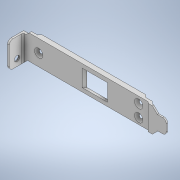
# Autodesk Inventor part: pcie-bracket
Saved by Autodesk Inventor 2021 (Build 250183000, 183)
## iProperties
Created: 2024-03-16
Part Number: pcie-bracket
Material: Generic
Document SubType Name: Modeling
Designer: Toby
Density: 1 g/cm^3
Appearance: Default
Author: Toby
Autodesk Inventor part; units mm, degrees
ref_plane "YZ Plane" through (0, 0, 0) normal (1, 0, 0) x (0, 1, 0)
ref_plane "XZ Plane" through (0, 0, 0) normal (0, 1, 0) x (-1, 0, 0)
ref_plane "XY Plane" through (0, 0, 0) normal (0, 0, 1) x (1, 0, 0)
sketch "Sketch1" plane through (0, 0, 0) normal (0, 0, 1) x (1, 0, 0)
  line L0 (-54.464, 10.0328) -> (58.286, 10.0328)
  line L1 (58.286, 10.0328) -> (58.286, -10.415)
  line L2 (58.286, -10.415) -> (-54.464, -10.415)
  line L3 (-54.464, -10.415) -> (-54.464, 10.0328)
  line L4 (58.286, 5.794) -> (65.556, 5.794)
  line L5 (65.556, 5.794) -> (65.556, -5.8813)
  line L6 (65.556, -5.8813) -> (58.286, -5.8813)
  line L7 (58.286, -5.8813) -> (58.286, 5.794)
  point P0 (0, 0)
  dimension "d0" = 112.75
  dimension "d1" = 120.02
  constraints: 16 end point, 4 parallel, 2 horizontal, 2 perpendicular, 1 point on line
  measures "d0" distance of L0.start L0.end
  measures "d1" distance between parallel lines of L3 L5
extrude "Extrusion1" add sketch "Sketch1" along normal blind 2
chamfer "Chamfer1" distance 4.2 angle 45 2 edges at (58.286, 10.0328, 1) (58.286, -10.415, 1)
fillet "Fillet1" radius 2 2 edges at (65.556, 5.794, 1) (65.556, -5.8813, 1)
sketch "Sketch3" plane through (-54.464, -10.415, 0) normal (-1, 0, 0) x (0, 0, 1)
  line L0 (0, 20.4479) -> (0, 0) projected
  line L1 (0, 17.9079) -> (13.43, 17.9079)
  line L2 (13.43, 17.9079) -> (13.43, -3.6821)
  line L3 (13.43, -3.6821) -> (0, -3.6821)
  line L4 (0, -3.6821) -> (0, 17.9079)
  line L5 (0, 20.4479) -> (2, 20.4479) projected
  line L6 (2, 20.4479) -> (2, 0) projected
  point P0 (0, 10.415)
  dimension "d14" = 2.54
  dimension "d15" = 21.59
  dimension "d16" = 11.43
  constraints: 8 end point, 2 parallel, 1 horizontal, 1 perpendicular, 1 point on line
  measures "d14" distance between parallel lines of L5 L1
  measures "d15" distance of L1.end L2.end
  measures "d16" distance between parallel lines of L2 L6
extrude "Extrusion3" add sketch "Sketch3" along normal blind 1.5 contours L1 L2 L3 L4 L0
sketch "Sketch4" plane through (0, 0, 0) normal (0, 0, -1) x (-1, 0, 0)
  line L0 (55.964, -14.0972) -> (55.964, 7.4928) projected
  line L1 (-54.086, 10.0328) -> (54.464, 10.0328) projected
  line L2 (55.964, 7.4928) -> (52.024, 7.4928)
  line L3 (52.024, 7.4928) -> (52.024, 10.0328)
  line L4 (52.024, 10.0328) -> (55.964, 10.0328)
  line L5 (55.964, 10.0328) -> (55.964, 7.4928)
  point P0 (0, 0)
  point P1 (-30.556, 10.0328)
  dimension "d19" = 3.94
  constraints: 8 end point, 2 parallel, 1 horizontal, 1 perpendicular, 1 point on line
  measures "d19" distance between parallel lines of L3 L5
extrude "Extrusion4" cut sketch "Sketch4" against normal blind 20
chamfer "Chamfer3" distance 2.54 angle 45 1 edges at (-52.024, 10.0328, 1)
chamfer "Chamfer4" distance 3.68 angle 45 1 edges at (-54.464, -10.415, 1)
fillet "Fillet2" radius 3 2 edges at (-55.214, 7.4928, 13.43) (-55.214, -14.0972, 13.43)
sketch "Sketch5" plane through (-55.964, -10.415, 0) normal (-1, 0, 0) x (0, 0, 1)
  circle A0 centre (7.08, 2.0279) radius 2.21
  line L0 (0, -3.6821) -> (10.43, -3.6821) projected
  line L1 (9.29, 2.0279) -> (4.87, 2.0279)
  line L2 (4.87, 2.0279) -> (4.87, -3.6821)
  line L3 (4.87, -3.6821) -> (9.29, -3.6821)
  line L4 (9.29, -3.6821) -> (9.29, 2.0279)
  line L5 (2, 20.4479) -> (0, 20.4479) projected
  line L6 (2, 17.9079) -> (2, 20.4479) projected
  point P0 (0, 10.415)
  point P1 (7.08, 2.0279)
  point P2 (9.29, -3.6821)
  point P3 (4.87, 2.0279)
  dimension "d29" = 4.42
  dimension "d30" = 18.42
  dimension "d31" = 5.08
  dimension "d32" = 5.08
  dimension "d33" = 4.42
  constraints: 8 end point, 2 parallel, 1 coincident, 1 horizontal, 1 midpoint, 1 perpendicular, 1 point on line, 3 other
  measures "d30" distance from line of L5 point (7.08, 2.028)
  measures "d31" distance from line of L6 point (7.08, 2.028)
  measures "d32" distance from line of L6 point (7.08, 2.028)
  measures "d33" distance between parallel lines of L2 L4
extrude "Extrusion5" cut sketch "Sketch5" against normal blind 2
fillet "Fillet3" radius 1 1 edges at (-54.464, -3.3011, 2)
fillet "Fillet4" radius 1 1 edges at (-55.964, -3.3022, 0)
sketch "Sketch13" plane through (0, 0, 0) normal (0, 0, -1) x (-1, 0, 0)
  line L0 (-1.036, 6.4328) -> (0.964, 6.4328)
  line L1 (0.964, 6.4328) -> (-0.036, 8.0328)
  line L2 (-0.036, 8.0328) -> (-1.036, 6.4328)
  line L3 (-54.086, 10.0328) -> (49.484, 10.0328) projected
  line L4 (54.964, 7.4928) -> (54.964, -14.0972) projected
  point P0 (0, 0)
  point P1 (-30.556, 10.0328)
  dimension "d84" = 2
  dimension "d85" = 1.6
  dimension "d86" = 1
  dimension "d87" = 2
  dimension "d88" = 55
  constraints: 6 end point, 1 horizontal
  measures "d84" distance of L0.end L0.start
  measures "d85" vertical distance of L0.end L1.end
  measures "d86" horizontal distance of L0.start L1.end
  measures "d87" distance from line of L3 L1.end
  measures "d88" distance from line of L4 L1.end
extrude "Extrusion12" cut sketch "Sketch13" against normal blind 0.4
sketch "Sketch14" plane through (0, 0, 2) normal (0, 0, 1) x (1, 0, 0)
  line L0 (-54.464, -11.0972) -> (-54.464, 4.4928) projected
  line L1 (-50.784, -10.415) -> (54.086, -10.415) projected
  line L2 (54.086, 10.0328) -> (-49.484, 10.0328) projected
  point P0 (0, 0)
  point P1 (-41.464, -0.415)
  point P2 (41.536, -5.415)
  point P3 (41.536, 4.585)
  dimension "d91" = 13
  dimension "d92" = 10
  dimension "d93" = 96
  dimension "d94" = 96
  dimension "d95" = 15
  dimension "d96" = 5
  dimension "d97" = 5.4479
  measures "d91" distance from line of L0 point (-41.464, -0.415)
  measures "d92" distance from line of L1 point (-41.464, -0.415)
  measures "d93" distance from line of L0 point (41.536, 4.585)
  measures "d94" distance from line of L0 point (41.536, -5.415)
  measures "d95" distance from line of L1 point (41.536, 4.585)
  measures "d96" distance from line of L1 point (41.536, -5.415)
  measures "d97" distance from line of point (41.536, 4.585) L2
hole "Hole2" at (-41.464, -0.415, 2) at (41.536, -5.415, 2) at (41.536, 4.585, 2) direction (0, 0, -1) diameter 3 depth 5 tip angle 118 countersink diameter 7 countersink angle 90
sketch "Sketch17" plane through (-49.484, 10.0328, 0) normal (0, 1, 0) x (1, 0, 0)
  line L0 (103.57, -2) -> (0, -2) projected
  line L1 (5.02, -2) -> (100.04, -2)
  line L2 (100.04, -2) -> (100.04, 2)
  line L3 (100.04, 2) -> (5.02, 2)
  line L4 (5.02, 2) -> (5.02, -2)
  line L5 (-4.98, -10.43) -> (-4.98, -3) projected
  line L6 (115.04, -2) -> (115.04, 0) projected
  point P0 (49.484, 0)
  dimension "d114" = 4
  dimension "d115" = 10
  dimension "d116" = 15
  constraints: 8 end point, 2 parallel, 1 horizontal, 1 perpendicular, 1 point on line
  measures "d114" distance between parallel lines of L0 L3
  measures "d115" distance between parallel lines of L5 L4
  measures "d116" distance from line of L6 L2.end
extrude "Extrusion14" add sketch "Sketch17" against normal blind 1.2
chamfer "Chamfer8" distance 2 angle 45 2 edges at (-44.464, 9.4328, -2) (50.556, 9.4328, -2)
sketch "Sketch18" plane through (0, 0, 2) normal (0, 0, 1) x (1, 0, 0)
  line L0 (-3.464, 6.385) -> (13.536, 6.385)
  line L1 (13.536, 6.385) -> (13.536, -6.815)
  line L2 (13.536, -6.815) -> (-3.464, -6.815)
  line L3 (-3.464, -6.815) -> (-3.464, 6.385)
  circle A0 centre (41.536, 4.585) radius 1.5 projected
  line L4 (-50.784, -10.415) -> (54.086, -10.415) projected
  point P0 (0, 0)
  dimension "d122" = 28
  dimension "d123" = 45
  dimension "d124" = 3.6
  dimension "d125" = 13.2
  constraints: 8 end point, 2 parallel, 1 horizontal, 1 perpendicular
  measures "d122" distance from line of A0.centre L1
  measures "d123" distance from line of A0.centre L3
  measures "d124" distance between parallel lines of L4 L2
  measures "d125" distance between parallel lines of L2 L0
extrude "Extrusion15" cut sketch "Sketch18" against normal blind 2 contours L0 L1 L2 L3
sketch "Sketch20" plane through (0, 0, 2) normal (0, 0, 1) x (1, 0, 0)
  line L0 (65.556, -5.8813) -> (58.286, -5.8813)
  line L1 (58.286, -5.8813) -> (58.286, 5.794)
  line L2 (58.286, 5.794) -> (65.556, 5.794)
  line L3 (65.556, 5.794) -> (65.556, -5.8813)
  line L4 (58.286, -10.415) -> (51.286, -10.415)
  line L5 (51.286, -10.415) -> (51.286, 10.0328)
  line L6 (51.286, 10.0328) -> (58.286, 10.0328)
  line L7 (58.286, 10.0328) -> (58.286, -10.415)
  line L8 (65.556, -3.8813) -> (65.556, 3.794) projected
  line L9 (58.286, -5.8813) -> (63.556, -5.8813) projected
  line L10 (63.556, 5.794) -> (58.286, 5.794) projected
  line L11 (54.086, 10.0328) -> (-49.484, 10.0328) projected
  line L12 (-50.784, -10.415) -> (54.086, -10.415) projected
  line L13 (58.286, -6.215) -> (58.286, -5.8813) projected
  point P0 (0, 0)
  dimension "d136" = 7
  constraints: 16 end point, 6 collinear, 4 parallel, 2 horizontal, 2 perpendicular, 1 point on line
  measures "d136" distance of L4.start L4.end
extrude "Extrusion17" add sketch "Sketch20" along normal blind 2
chamfer "Chamfer11" distance 4.2 angle 45 2 edges at (58.286, -10.415, 3) (58.286, 10.0328, 3)
chamfer "Chamfer12" distance 2 angle 45 1 edges at (51.286, -0.1911, 2)
sketch "Sketch21" plane through (-50.784, -10.415, 0) normal (0, -1, 0) x (1, 0, 0)
  line L0 (116.34, 0) -> (114.34, 0) projected
  line L1 (116.34, 0) -> (103.34, 0)
  line L2 (103.34, 0) -> (103.34, 2)
  line L3 (103.34, 2) -> (116.34, 2)
  line L4 (116.34, 2) -> (116.34, 0)
  line L5 (114.34, 2) -> (116.34, 2) projected
  line L6 (104.87, 0) -> (101.34, 0) projected
  point P0 (50.784, 0)
  dimension "d145" = 2
  constraints: 8 end point, 2 parallel, 1 collinear, 1 horizontal, 1 perpendicular
  measures "d145" distance from line of L2 L6.end
extrude "Extrusion18" cut sketch "Sketch21" against normal blind 200
chamfer "Chamfer13" distance 2 angle 45 1 edges at (52.556, -0.1911, 0)
fillet "Fillet10" radius 3 2 edges at (65.556, -5.8813, 3) (65.556, 5.794, 3)
sketch "Sketch22" plane through (-50.784, -10.415, 0) normal (0, -1, 0) x (1, 0, 0)
  line L0 (101.14, 4) -> (116.34, 4)
  line L1 (116.34, 4) -> (116.34, 3.2)
  line L2 (116.34, 3.2) -> (101.14, 3.2)
  line L3 (101.14, 3.2) -> (101.14, 4)
  line L4 (102.07, 4) -> (104.87, 4) projected
  line L5 (116.34, 2) -> (116.34, 4) projected
  point P0 (50.784, 0)
  dimension "d152" = 15.2
  dimension "d153" = 0.8
  constraints: 8 end point, 2 collinear, 2 parallel, 1 horizontal, 1 perpendicular
  measures "d152" distance between parallel lines of L1 L3
  measures "d153" distance between parallel lines of L0 L2
extrude "Extrusion19" cut sketch "Sketch22" against normal blind 200
sketch "Sketch23" plane through (-49.484, 8.8328, 0) normal (0, -1, 0) x (1, 0, 0)
  line L0 (5.02, 0) -> (100.04, 0) projected
  line L1 (7.02, -2) -> (98.04, -2) projected
  line L2 (100.04, 0) -> (95.04, 0)
  line L3 (95.04, 0) -> (95.04, -2)
  line L4 (95.04, -2) -> (100.04, -2)
  line L5 (100.04, -2) -> (100.04, 0)
  point P0 (49.484, 0)
  dimension "d156" = 5
  constraints: 8 end point, 2 parallel, 1 horizontal, 1 perpendicular, 1 point on line
  measures "d156" distance between parallel lines of L5 L3
extrude "Extrusion20" cut sketch "Sketch23" against normal blind 10
chamfer "Chamfer14" distance 2 angle 45 1 edges at (45.556, 9.4328, -2)
sketch "Sketch24" plane through (-55.964, -10.415, 0) normal (-1, 0, 0) x (0, 0, 1)
  arc A0 (9.29, 2.0279) -> (4.87, 2.0279) centre (7.08, 2.0279) ccw projected
  circle A1 centre (7.08, 2.0279) radius 2.21
  line L0 (4.87, -3.6821) -> (4.87, 2.0279) projected
  line L1 (9.29, 2.0279) -> (9.29, -3.6821) projected
  line L2 (4.87, -3.6821) -> (9.29, -3.6821)
  line L3 (9.29, -3.6821) -> (9.29, -0.6821)
  line L4 (9.29, -0.6821) -> (4.87, -0.6821)
  line L5 (4.87, -0.6821) -> (4.87, -3.6821)
  point P0 (0, 10.415)
  point P1 (9.29, 2.0279)
  point P2 (4.87, 2.0279)
  dimension "d162" = 3
  constraints: 8 end point, 2 coincident, 2 parallel, 1 centre point, 1 concentric, 1 horizontal, 1 perpendicular, 1 point on line
  measures "d162" distance between parallel lines of L2 L4
extrude "Extrusion21" add sketch "Sketch24" against normal blind 1.5 contours L1 L4 L0 A1 | L1 L2 L0 L4
chamfer "Chamfer15" distance 0.4 angle 45 2 edges at (-55.964, -10.5972, 7.08) (-55.964, -6.1772, 7.08)
sketch "Sketch25" plane through (0, 0, 2) normal (0, 0, 1) x (1, 0, 0)
  line L0 (13.536, -7.215) -> (-3.464, -7.215)
  line L1 (-3.464, -7.215) -> (-3.464, 6.785)
  line L2 (-3.464, 6.785) -> (13.536, 6.785)
  line L3 (13.536, 6.785) -> (13.536, -7.215)
  line L4 (13.536, 6.385) -> (13.536, -6.815) projected
  line L5 (-3.464, -6.815) -> (-3.464, 6.385) projected
  line L6 (13.536, -6.815) -> (-3.464, -6.815) projected
  line L7 (-3.464, 6.385) -> (13.536, 6.385) projected
  point P0 (0, 0)
  dimension "d168" = 0.4
  dimension "d169" = 0.4
  constraints: 8 end point, 2 collinear, 2 parallel, 1 horizontal, 1 perpendicular
  measures "d168" distance between parallel lines of L6 L0
  measures "d169" distance between parallel lines of L2 L7
extrude "Extrusion22" cut sketch "Sketch25" against normal blind 2
chamfer "Chamfer16" distance 2 angle 45 6 edges at (13.536, -7.015, 2) (13.536, -0.215, 2) (13.536, 6.585, 2) (-3.464, -0.215, 2) (-3.464, -7.015, 2) (-3.464, 6.585, 2)
body "Solid1"
